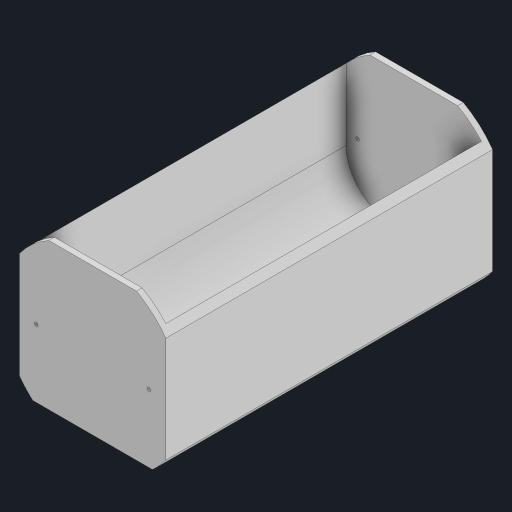
# Autodesk Inventor part: CAJA PARA DETECCION DE OBJETO
Saved by Autodesk Inventor 2024.3 (Build 283343000, 343)
## iProperties
Created: 2024-06-16
Part Number: CAJA PARA DETECCION DE OBJETO
Material: Generic
Document SubType Name: Modeling
Designer: Jhuliams
Density: 1 g/cm^3
Appearance: Default
Author: Jhuliams
Autodesk Inventor part; units mm, degrees
ref_plane "YZ Plane" through (0, 0, 0) normal (1, 0, 0) x (0, 1, 0)
ref_plane "XZ Plane" through (0, 0, 0) normal (0, 1, 0) x (-1, 0, 0)
sketch "Sketch1" plane through (0, 0, 0) normal (0, 1, 0) x (-1, 0, 0)
  line L0 (65, 145) -> (-65, 145)
  line L1 (-65, 145) -> (-65, -145)
  line L2 (-65, -145) -> (65, -145)
  line L3 (65, -145) -> (65, 145)
  line L4 (65, 145) -> (-65, -145) construction
  line L5 (-65, 145) -> (65, -145) construction
  point P0 (0, 0)
  dimension "d0" = 130
  dimension "d1" = 290
  constraints: 12 end point, 2 midpoint, 2 parallel, 1 horizontal, 1 perpendicular
  measures "d0" distance of L2.end L1.end
  measures "d1" distance of L1.end L0.end
extrude "Extrusion1" add sketch "Sketch1" along normal blind 130
sketch "Sketch2" plane through (0, 130, 0) normal (0, 1, 0) x (1, 0, 0)
  line L0 (-60, 140) -> (60, 140)
  line L1 (60, 140) -> (60, -140)
  line L2 (60, -140) -> (-60, -140)
  line L3 (-60, -140) -> (-60, 140)
  line L4 (-60, 140) -> (60, -140) construction
  line L5 (60, 140) -> (-60, -140) construction
  point P0 (0, 0)
  dimension "d4" = 120
  dimension "d5" = 280
  constraints: 12 end point, 2 midpoint, 2 parallel, 1 horizontal, 1 perpendicular
  measures "d4" distance of L1.end L2.end
  measures "d5" distance of L0.end L1.end
extrude "Extrusion2" cut sketch "Sketch2" against normal blind 120
ref_plane "Work Plane1" through (0, 60, 0) normal (0, 1, 0) x (1, 0, 0)
sketch "Sketch3" plane through (0, 60, 0) normal (0, 1, 0) x (1, 0, 0)
  line L0 (-65, 145) -> (-65, -145) projected
  line L1 (65, -145) -> (65, 145) projected
  line L2 (-65, 0) -> (-80, 0)
  line L3 (-80, 0) -> (-80, 150)
  line L4 (-80, 150) -> (-70, 150)
  line L5 (0, 0) -> (0, 46.0375) construction
  line L6 (65, 0) -> (80, 0)
  line L7 (80, 0) -> (80, 152.0021)
  line L8 (70, 145) -> (65, 0)
  line L9 (65, 145) -> (-65, 145) construction
  line L10 (-30.0305, 159.5477) -> (0, 170.4779)
  line L11 (-65, 145) -> (26.4544, 145) construction
  line L12 (65, 145) -> (161.3863, 145) construction
  line L13 (0, 181.1197) -> (-80, 152.0021)
  line L14 (0, 181.1197) -> (80, 152.0021)
  line L15 (30.0305, 159.5477) -> (0, 170.4779)
  line L16 (-14.619, 175.7988) -> (-15.875, 176.2559)
  line L17 (-70, 150) -> (-70, 155.6418)
  line L18 (-65, 145) -> (-65, 0)
  arc A0 (-30.0305, 159.5477) -> (-27.4654, 145) centre (-27.4654, 152.5) ccw
  arc A1 (27.4654, 145) -> (30.0305, 159.5477) centre (27.4654, 152.5) ccw
  line L19 (27.4654, 145) -> (-27.4654, 145)
  line L20 (-65, 145) -> (-27.4654, 145)
  line L21 (27.4654, 145) -> (70, 145)
  line L22 (0, 0) -> (30, 0) construction
  line L23 (-80, 0) -> (-80, -150)
  line L24 (-80, -150) -> (-70, -150)
  line L25 (0, 0) -> (0, -46.0375) construction
  line L26 (80, 0) -> (80, -152.0021)
  line L27 (70, -145) -> (65, 0)
  line L28 (65, -145) -> (-65, -145) construction
  line L29 (-30.0305, -159.5477) -> (0, -170.4779)
  line L30 (-65, -145) -> (26.4544, -145) construction
  line L31 (65, -145) -> (161.3863, -145) construction
  line L32 (0, -181.1197) -> (-80, -152.0021)
  line L33 (0, -181.1197) -> (80, -152.0021)
  line L34 (30.0305, -159.5477) -> (0, -170.4779)
  line L35 (-14.619, -175.7988) -> (-15.875, -176.2559)
  line L36 (-70, -150) -> (-70, -155.6418)
  line L37 (-65, -145) -> (-65, 0)
  arc A2 (-27.4654, -145) -> (-30.0305, -159.5477) centre (-27.4654, -152.5) ccw
  arc A3 (30.0305, -159.5477) -> (27.4654, -145) centre (27.4654, -152.5) ccw
  line L38 (27.4654, -145) -> (-27.4654, -145)
  line L39 (-65, -145) -> (-27.4654, -145)
  line L40 (27.4654, -145) -> (70, -145)
  point P0 (70, 150)
  point P1 (65, 0)
  point P2 (70, -150)
  dimension "d9" = 10
  dimension "d10" = 150
  dimension "d11" = 20
  dimension "d13" = 10
  dimension "d15" = 15
  dimension "d33" = 30
  constraints: 76 end point, 25 symmetric about line, 12 point on line, 8 point on circle, 4 centre point, 4 horizontal, 3 parallel, 3 tangent, 2 collinear, 1 midpoint, 1 perpendicular, 1 vertical, 3 other
  measures "d9" distance of L3.end L4.end
  measures "d10" distance of L2.end L3.end
  measures "d11" angle of L11 L10
  measures "d13" distance between parallel lines of L10 L13
  measures "d15" diameter of A0
  measures "d33" distance of L5.start L22.end
extrude "Extrusion3" add sketch "Sketch3" along normal mid plane 40 contours L0 L2 L3 L4 L17 L13 L14 L7 L6 L8 L21 A1 L15 L10 A0 L20 | L0 L39 A2 L29 L34 A3 L40 L27 L6 L26 L33 L32 L36 L24 L23 L2 | L21 L8 L1
ref_plane "Work Plane2" through (0, 0, -186.12) normal (0, 0, 1) x (1, 0, 0)
sketch "Sketch5" plane through (0, 0, -186.12) normal (0, 0, 1) x (1, 0, 0)
  line L0 (0, 0) -> (0, 60)
  line L1 (0, 40) -> (0, 80) projected
  circle A0 centre (0, 60) radius 10
  dimension "d21" = 60
  dimension "d22" = 20
  constraints: 2 end point, 1 centre point, 1 coincident, 1 midpoint
  measures "d21" distance of L0.start L0.end
  measures "d22" diameter of A0
extrude "Extrusion4" add sketch "Sketch5" along normal blind 30
fillet "Fillet2" radius 5 3 edges at (7.0711, 52.9289, -178.546) (7.0711, 67.0711, -178.546) (-10, 60, -177.48)
sketch "Sketch6" plane through (0, 60, -186.12) normal (0, 0, -1) x (-1, 0, 0)
  line L0 (-3, 12.5) -> (3, 12.5)
  line L1 (3, 12.5) -> (3, -12.5)
  line L2 (3, -12.5) -> (-3, -12.5)
  line L3 (-3, -12.5) -> (-3, 12.5)
  line L4 (0, -20) -> (0, 20) projected
  line L5 (-3, 12.5) -> (3, -12.5) construction
  line L6 (3, 12.5) -> (-3, -12.5) construction
  arc A0 (-2.3337, 9.7239) -> (2.3337, 9.7239) centre (0, 0) ccw
  line L7 (3, 9.5394) -> (3, 4.0784)
  line L8 (3, 4.0784) -> (-3, 4.0784)
  line L9 (-3, 4.0784) -> (-3, 9.5394)
  line L10 (-3, 9.5394) -> (-2.2895, 9.5394)
  line L11 (2.2895, 9.5394) -> (3, 9.5394)
  line L12 (-3, 9.5394) -> (-2.2895, 9.5394)
  point P0 (0, -60)
  point P1 (3, 4.0784)
  point P2 (-3, 4.0784)
  dimension "d26" = 6
  dimension "d27" = 25
  dimension "d28" = 20
  dimension "d29" = 6
  dimension "d30" = 5.461
  constraints: 24 end point, 5 parallel, 5 point on line, 3 horizontal, 3 midpoint, 3 perpendicular, 3 point on circle, 1 centre point, 1 coincident
  measures "d26" distance of L1.end L2.end
  measures "d27" distance of L0.end L1.end
  measures "d28" diameter of A0
  measures "d29" distance of L7.end L8.end
  measures "d30" distance of L7.start L7.end
extrude "Extrusion5" cut sketch "Sketch6" along normal mid plane 20 contours L0 L4 L8 L3 | L0 L1 L8 L4
sketch "Sketch7" plane through (0, 0, -186.12) normal (0, 0, -1) x (-1, 0, 0)
  arc A0 (-3, 69.5394) -> (3, 69.5394) centre (0, 60) ccw projected
  circle A1 centre (0, 60) radius 10
  point P0 (0, 0)
  point P1 (3, 69.5394)
  constraints: 1 centre point, 1 coincident, 1 concentric
extrude "Extrusion6" add sketch "Sketch7" along normal blind 20
mirror "Mirror1" about plane through (0, 0, 0) normal (0, 0, 1) of "Extrusion4"
fillet "Fillet3" radius 5 3 edges at (7.0711, 52.9289, 178.546) (7.0711, 67.0711, 178.546) (-10, 60, 177.48)
sketch "Sketch8" plane through (-65, 0, 145) normal (0, 0, 1) x (1, 0, 0)
  line L0 (37.5346, 80) -> (37.5346, 40) projected
  line L1 (0, 0) -> (0, 40) projected
  line L2 (0, 0) -> (130, 0) projected
  line L3 (130, 0) -> (130, 40) projected
  line L4 (92.4654, 80) -> (92.4654, 40) projected
  line L5 (130, 80) -> (130, 130) projected
  line L6 (0, 130) -> (130, 130) projected
  line L7 (0, 80) -> (0, 130) projected
  line L8 (42.5346, 40) -> (97.4654, 100)
  arc A0 (62, 69.5394) -> (64.4128, 50.0173) centre (65, 60) ccw projected
  circle A1 centre (65, 60) radius 80.106
  line L9 (0, 80) -> (37.5346, 80) projected
  line L10 (37.5346, 40) -> (0, 40) projected
  line L11 (130, 40) -> (92.4654, 40) projected
  line L12 (92.4654, 80) -> (130, 80) projected
  point P0 (65, 0)
  point P1 (62.5464, 76.6667)
  point P2 (62.5464, 63.3333)
  point P3 (103.9483, 130)
  point P4 (130, 106.8185)
  point P5 (0, 106.8185)
  point P6 (26.0517, 130)
  constraints: 2 end point, 1 centre point, 1 coincident
extrude "Extrusion7" cut sketch "Sketch8" against normal through all contours L7 L6 A1 | L6 L5 A1
sketch "Sketch9" plane through (-65, 0, 145) normal (0, 0, 1) x (1, 0, 0)
  line L0 (-190.4665, 210.1855) -> (344.6841, 210.1855)
  line L1 (344.6841, 210.1855) -> (344.6841, -61.655)
  line L2 (344.6841, -61.655) -> (-190.4665, -61.655)
  line L3 (-190.4665, -61.655) -> (-190.4665, 210.1855)
  point P0 (65, 0)
  constraints: 8 end point, 2 parallel, 1 horizontal, 1 perpendicular
extrude "Extrusion8" cut sketch "Sketch9" along normal through all
sketch "Sketch10" plane through (65, 0, -145) normal (0, 0, -1) x (-1, 0, 0)
  line L0 (-91.2878, 177.5286) -> (271.6098, 177.5286)
  line L1 (271.6098, 177.5286) -> (271.6098, -56.5627)
  line L2 (271.6098, -56.5627) -> (-91.2878, -56.5627)
  line L3 (-91.2878, -56.5627) -> (-91.2878, 177.5286)
  point P0 (65, 0)
  constraints: 8 end point, 2 parallel, 1 horizontal, 1 perpendicular
extrude "Extrusion9" cut sketch "Sketch10" along normal through all
sketch "Sketch11" plane through (-65, 0, 145) normal (0, 0, 1) x (1, 0, 0)
  line L0 (130, 0) -> (130, 106.8185) projected
  arc A0 (130, 106.8185) -> (103.9483, 130) centre (65, 60) ccw projected
  line L1 (26.0517, 130) -> (103.9483, 130) projected
  arc A1 (26.0517, 130) -> (0, 106.8185) centre (65, 60) ccw projected
  line L2 (0, 80) -> (0, 106.8185) projected
  line L3 (-15, 40) -> (-15, 80) projected
  line L4 (0, 0) -> (0, 40) projected
  line L5 (0, 0) -> (130, 0) projected
  circle A2 centre (15, 60) radius 1.5
  line L6 (65, 60) -> (65, 81.4115)
  line L7 (5, 113.0752) -> (5, 10) projected
  line L8 (5, 113.0752) -> (5, 10) projected
  circle A3 centre (115, 60) radius 1.5
  line L9 (-15, 80) -> (0, 80) projected
  line L10 (0, 40) -> (-15, 40) projected
  point P0 (65, 0)
  point P1 (-15, 60)
  dimension "d43" = 3
  dimension "d45" = 30
  constraints: 2 centre point, 2 end point, 1 horizontal alignment, 1 midpoint, 1 symmetric about line, 1 vertical, 1 other
  measures "d43" diameter of A2
  measures "d45" distance from line of A2.centre L3
extrude "Extrusion10" cut sketch "Sketch11" against normal through all contours A2 | A3
sketch "Sketch17" plane through (65, 0, -145) normal (0, 0, -1) x (-1, 0, 0)
  circle A0 centre (15, 60) radius 1.5 projected
  circle A1 centre (115, 60) radius 1.5 projected
  arc A2 (26.0517, 130) -> (0, 106.8185) centre (65, 60) ccw projected
  line L0 (0, 80) -> (0, 106.8185) projected
  line L1 (-15, 40) -> (-15, 80) projected
  line L2 (0, 0) -> (0, 40) projected
  line L3 (0, 0) -> (130, 0) projected
  line L4 (130, 0) -> (130, 40) projected
  line L5 (145, 80) -> (145, 40) projected
  line L6 (130, 80) -> (130, 106.8185) projected
  arc A3 (130, 106.8185) -> (103.9483, 130) centre (65, 60) ccw projected
  line L7 (26.0517, 130) -> (103.9483, 130) projected
  line L8 (130, 0) -> (130, 106.8185)
  line L9 (0, 0) -> (0, 106.8185)
  line L10 (-15, 80) -> (0, 80) projected
  line L11 (0, 40) -> (-15, 40) projected
  line L12 (145, 40) -> (130, 40) projected
  line L13 (130, 80) -> (145, 80) projected
  point P0 (65, 0)
  point P1 (0, 40)
  point P2 (0, 80)
  point P3 (130, 80)
  point P4 (130, 40)
  constraints: 4 end point, 1 collinear, 1 vertical
extrude "Extrusion16" cut sketch "Sketch17" against normal through all contours L9 L11 L1 L10 | L13 L5 L12 L8
fillet "Fillet4" radius 40 2 edges at (60, 10, 0) (-60, 10, 0)
sketch "Sketch18" plane through (65, 0, -145) normal (0, 0, -1) x (-1, 0, 0)
  line L0 (0, 0) -> (0, 106.8185) projected
  line L1 (0, 0) -> (130, 0) projected
  line L2 (130, 0) -> (130, 106.8185) projected
  arc A0 (130, 106.8185) -> (103.9483, 130) centre (65, 60) ccw projected
  line L3 (26.0517, 130) -> (103.9483, 130) projected
  arc A1 (26.0517, 130) -> (0, 106.8185) centre (65, 60) ccw projected
  circle A2 centre (15, 60) radius 1.5 projected
  circle A3 centre (115, 60) radius 1.5 projected
  circle A4 centre (65, 60) radius 80.106
  circle A5 centre (15, 60) radius 1.5 projected
  circle A6 centre (115, 60) radius 1.5 projected
  line L4 (85, 10) -> (45, 10) projected
  arc A7 (26.0517, 130) -> (5, 113.0752) centre (65, 60) ccw projected
  line L5 (103.9483, 130) -> (26.0517, 130) projected
  arc A8 (125, 113.0752) -> (103.9483, 130) centre (65, 60) ccw projected
  arc A9 (85, 10) -> (125, 50) centre (85, 50) ccw projected
  arc A10 (5, 50) -> (45, 10) centre (45, 50) ccw projected
  line L6 (5, 113.0752) -> (5, 50) projected
  line L7 (125, 113.0752) -> (125, 50) projected
  point P0 (65, 0)
  point P1 (130, 13.1815)
  point P2 (118.0752, 0)
  point P3 (11.9248, 0)
  point P4 (0, 13.1815)
  constraints: 1 centre point, 1 coincident, 1 concentric
extrude "Extrusion17" cut sketch "Sketch18" against normal through all contours L0 A4 L1 | A4 L2 L1
sketch "Sketch12" plane through (-65, 0, 145) normal (0, 0, 1) x (1, 0, 0)
  line L0 (-71.3977, 197.918) -> (200.9094, 197.918)
  line L1 (200.9094, 197.918) -> (200.9094, -42.9243)
  line L2 (200.9094, -42.9243) -> (-71.3977, -42.9243)
  line L3 (-71.3977, -42.9243) -> (-71.3977, 197.918)
  point P0 (65, 0)
  dimension "d50" = 5
  dimension "d62" = 0.25
  constraints: 40 end point, 24 point on circle, 12 centre point, 30 other
sketch "Sketch14" plane through (0, 0, 0) normal (0, 0, 1) x (1, 0, 0)
  line L0 (-82.5, 44.3301) -> (-85, 45) projected
  arc A0 (-75, 40) -> (-82.5, 44.3301) centre (-80, 40) ccw projected
  line L1 (-75, 40) -> (-75, 0) projected
  line L2 (-70, -5) -> (-75, 0) projected
  line L3 (-70, -5) -> (70, -5) projected
  line L4 (75, 0) -> (70, -5) projected
  line L5 (75, 0) -> (75, 40) projected
  arc A1 (82.5, 44.3301) -> (75, 40) centre (80, 40) ccw projected
  line L6 (85, 45) -> (82.5, 44.3301) projected
  line L7 (85, 45) -> (85, 95) projected
  line L8 (82.5, 95.6699) -> (85, 95) projected
  arc A2 (75, 100) -> (82.5, 95.6699) centre (80, 100) ccw projected
  line L9 (75, 100) -> (75, 110.2248) projected
  arc A3 (75, 110.2248) -> (63.4409, 126.7299) centre (0, 70) ccw projected
  line L10 (60, 125.3575) -> (63.4409, 126.7299) projected
  line L11 (60, 125.3575) -> (60, 20) projected
  line L12 (55, 15) -> (60, 20) projected
  line L13 (55, 15) -> (-55, 15) projected
  line L14 (-60, 20) -> (-55, 15) projected
  line L15 (-60, 20) -> (-60, 125.3575) projected
  line L16 (-63.4409, 126.7299) -> (-60, 125.3575) projected
  arc A4 (-63.4409, 126.7299) -> (-75, 110.2248) centre (0, 70) ccw projected
  line L17 (-75, 110.2248) -> (-75, 100) projected
  arc A5 (-82.5, 95.6699) -> (-75, 100) centre (-80, 100) ccw projected
  line L18 (-85, 95) -> (-82.5, 95.6699) projected
  line L19 (-85, 95) -> (-85, 45) projected
  point P0 (0, 0)
body "Solid1"
